Autodesk Fusion 360 part; units mm, degrees
(part 2 of 2)
sketch "Sketch1" plane through (0, 0, 0) normal (0, 0, 1) x (1, 0, 0)
  line L0 (-42.9407, 21.9767) -> (-42.9407, 26.9767)
  line L1 (-42.9407, 26.9767) -> (-52.9407, 26.9767)
  line L2 (-52.9407, 26.9767) -> (-52.9407, 31.9767)
  line L3 (-52.9407, 31.9767) -> (-47.9407, 31.9767)
  line L4 (-47.9407, 31.9767) -> (-47.9407, 41.9767)
  line L5 (-47.9407, 41.9767) -> (-52.9407, 41.9767)
  line L6 (-32.9407, 26.9767) -> (-32.9407, 21.9767)
  line L7 (-22.9407, 26.9767) -> (-32.9407, 26.9767)
  line L8 (-22.9407, 21.9767) -> (-22.9407, 26.9767)
  line L9 (-12.9407, 26.9767) -> (-12.9407, 21.9767)
  line L10 (-2.9407, 26.9767) -> (-12.9407, 26.9767)
  line L11 (-27.9407, 12.4409) -> (-27.9407, 59.643) construction
  line L12 (-59.1616, 36.9767) -> (4.5103, 36.9767) construction
  line L13 (-42.9407, 46.9767) -> (-52.9407, 46.9767)
  line L14 (-42.9407, 51.9767) -> (-42.9407, 46.9767)
  line L15 (-32.9407, 46.9767) -> (-32.9407, 51.9767)
  line L16 (-22.9407, 46.9767) -> (-32.9407, 46.9767)
  line L17 (-22.9407, 51.9767) -> (-22.9407, 46.9767)
  line L18 (-12.9407, 46.9767) -> (-12.9407, 51.9767)
  line L19 (-2.9407, 46.9767) -> (-12.9407, 46.9767)
  line L20 (-7.9407, 31.9767) -> (-7.9407, 41.9767)
  line L21 (-7.9407, 41.9767) -> (-2.9407, 41.9767)
  line L22 (-2.9407, 31.9767) -> (-7.9407, 31.9767)
  line L23 (-42.9407, 51.9767) -> (-32.9407, 51.9767)
  line L24 (-22.9407, 51.9767) -> (-12.9407, 51.9767)
  line L25 (-52.9407, 26.9767) -> (-52.9407, 31.9767)
  line L26 (-52.9407, 41.9767) -> (-52.9407, 46.9767)
  line L27 (-12.9407, 21.9767) -> (-22.9407, 21.9767)
  line L28 (-32.9407, 21.9767) -> (-42.9407, 21.9767)
  line L29 (-2.9407, 46.9767) -> (-2.9407, 41.9767)
  line L30 (-2.9407, 31.9767) -> (-2.9407, 26.9767)
  dimension "d5" = 5
  dimension "d6" = 5
  dimension "d7" = 10
  dimension "d12" = 15
  dimension "d13" = 25
  constraint horizontal L23
  constraint vertical L29
  constraint horizontal L27
  constraint vertical L25
  constraint vertical L0
  constraint horizontal L1
  constraint perpendicular L1 L2
  constraint horizontal L3
  constraint vertical L4
  constraint horizontal L5
  constraint perpendicular L11 L23
  constraint perpendicular L12 L29
  constraint symmetric L0.start L12 L14.start
  constraint symmetric L0.end L12 L13.start
  constraint symmetric L1.end L12 L13.end
  constraint symmetric L6.start L12 L15.start
  constraint symmetric L6.end L12 L15.end
  constraint symmetric L7.start L12 L16.start
  constraint symmetric L8.start L12 L17.start
  constraint symmetric L9.start L12 L18.start
  constraint symmetric L9.end L12 L18.end
  constraint symmetric L10.start L12 L19.start
  constraint symmetric L2.end L11 L22.start
  constraint symmetric L3.end L11 L20.start
  constraint symmetric L4.end L11 L20.end
  constraint symmetric L5.end L11 L21.end
  constraint collinear L23 L24
  constraint collinear L25 L26
  constraint collinear L27 L28
  constraint collinear L29 L30
  measures "d5" distance of L1.end L2.end
  measures "d6" distance of L2.end L3.end
  measures "d7" distance of L2.end L5.end
  measures "d12" distance of L12 L23
  measures "d13" distance of L11 L29
extrude "Extrude1" add sketch "Sketch1" along normal blind 5
sketch "Sketch2" plane through (0, 0, 5) normal (0, 0, 1) x (-1, 0, 0)
  line L0 (7.9407, -31.9767) -> (7.9407, -41.9767)
  line L1 (7.9407, -41.9767) -> (2.9407, -41.9767)
  line L2 (2.9407, -41.9767) -> (2.9407, -46.9767)
  line L3 (2.9407, -46.9767) -> (12.9407, -46.9767)
  line L4 (12.9407, -46.9767) -> (12.9407, -51.9767)
  line L5 (12.9407, -51.9767) -> (22.9407, -51.9767)
  line L6 (22.9407, -51.9767) -> (22.9407, -46.9767)
  line L7 (22.9407, -46.9767) -> (32.9407, -46.9767)
  line L8 (32.9407, -46.9767) -> (32.9407, -51.9767)
  line L9 (32.9407, -51.9767) -> (42.9407, -51.9767)
  line L10 (42.9407, -51.9767) -> (42.9407, -46.9767)
  line L11 (42.9407, -46.9767) -> (52.9407, -46.9767)
  line L12 (52.9407, -46.9767) -> (52.9407, -41.9767)
  line L13 (52.9407, -41.9767) -> (47.9407, -41.9767)
  line L14 (47.9407, -41.9767) -> (47.9407, -31.9767)
  line L15 (47.9407, -31.9767) -> (52.9407, -31.9767)
  line L16 (52.9407, -31.9767) -> (52.9407, -26.9767)
  line L17 (52.9407, -26.9767) -> (42.9407, -26.9767)
  line L18 (42.9407, -26.9767) -> (42.9407, -21.9767)
  line L19 (42.9407, -21.9767) -> (32.9407, -21.9767)
  line L20 (32.9407, -21.9767) -> (32.9407, -26.9767)
  line L21 (32.9407, -26.9767) -> (22.9407, -26.9767)
  line L22 (22.9407, -26.9767) -> (22.9407, -21.9767)
  line L23 (22.9407, -21.9767) -> (12.9407, -21.9767)
  line L24 (12.9407, -21.9767) -> (12.9407, -26.9767)
  line L25 (12.9407, -26.9767) -> (2.9407, -26.9767)
  line L26 (2.9407, -26.9767) -> (2.9407, -31.9767)
  line L27 (2.9407, -31.9767) -> (7.9407, -31.9767)
  line L28 (43.5617, -39.2983) -> (32.0803, -39.2983) construction
  line L29 (32.0803, -39.2983) -> (32.0803, -43.9251) construction
  line L30 (32.0803, -43.9251) -> (43.5617, -43.9251) construction
  line L31 (43.5617, -43.9251) -> (43.5617, -39.2983) construction
  dimension "d16" = 5
  text T0 "1068" font "Arial" height 5 align left top in box 11.4814 x 4.6268 at (43.5617, -39.2983) x (-1, 0) y (0, -1) spacing 1 kerned
emboss "Emboss1" depth -0.7 profiles "Sketch2" section 1 text T0 onto face at (-39.6074, 33.6433, 5)

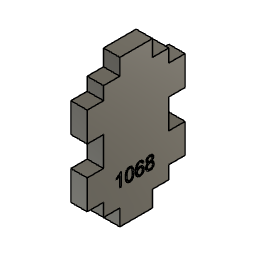
design "Housing_6"
Autodesk Fusion 360 part; units mm, degrees
sketch "Sketch1" plane through (0, 0, 0) normal (1, 0, 0) x (0, 1, 0)
  line L0 (-14.2005, 65.0328) -> (-4.2005, 65.0328)
  line L1 (-19.2005, 60.0328) -> (-19.2005, 56.0328)
  line L2 (-19.2005, 56.0328) -> (-24.2005, 56.0328)
  line L3 (-14.2005, 65.0328) -> (-14.2005, 60.0328)
  line L4 (-14.2005, 60.0328) -> (-19.2005, 60.0328)
  line L5 (-19.2005, 38.0328) -> (-24.2005, 38.0328)
  line L6 (-19.2005, 42.5328) -> (-19.2005, 38.0328)
  line L7 (-19.2005, 42.5328) -> (-19.2005, 47.0328)
  line L8 (-24.2005, 47.0328) -> (-19.2005, 47.0328)
  line L9 (-19.2005, 25.0328) -> (-19.2005, 27.5328)
  line L10 (-9.2005, 80.7683) -> (-9.2005, 14.0865) construction
  line L11 (-40.7163, 42.5328) -> (11.7648, 42.5328) construction
  line L12 (-4.2005, 60.0328) -> (0.7995, 60.0328)
  line L13 (-4.2005, 65.0328) -> (-4.2005, 60.0328)
  line L14 (0.7995, 60.0328) -> (0.7995, 56.0328)
  line L15 (0.7995, 56.0328) -> (5.7995, 56.0328)
  line L16 (5.7995, 47.0328) -> (0.7995, 47.0328)
  line L17 (0.7995, 42.5328) -> (0.7995, 47.0328)
  line L18 (0.7995, 42.5328) -> (0.7995, 38.0328)
  line L19 (0.7995, 38.0328) -> (5.7995, 38.0328)
  line L20 (-14.2005, 25.0328) -> (-19.2005, 25.0328)
  line L21 (-14.2005, 20.0328) -> (-14.2005, 25.0328)
  line L22 (-19.2005, 25.0328) -> (-19.2005, 29.0328)
  line L23 (-19.2005, 29.0328) -> (-24.2005, 29.0328)
  line L24 (-4.2005, 20.0328) -> (-4.2005, 25.0328)
  line L25 (-4.2005, 25.0328) -> (0.7995, 25.0328)
  line L26 (0.7995, 25.0328) -> (0.7995, 29.0328)
  line L27 (0.7995, 29.0328) -> (5.7995, 29.0328)
  line L28 (5.7995, 56.0328) -> (5.7995, 47.0328)
  line L29 (5.7995, 38.0328) -> (5.7995, 29.0328)
  line L30 (-4.2005, 20.0328) -> (-14.2005, 20.0328)
  line L31 (-24.2005, 29.0328) -> (-24.2005, 38.0328)
  line L32 (-24.2005, 47.0328) -> (-24.2005, 56.0328)
  line L33 (-4.2005, 65.0328) -> (-4.2005, 60.0328)
  line L34 (-4.2005, 60.0328) -> (0.7995, 60.0328)
  line L35 (0.7995, 56.0328) -> (5.7995, 56.0328)
  line L36 (0.7995, 60.0328) -> (0.7995, 56.0328)
  line L37 (5.7995, 47.0328) -> (5.7995, 56.0328)
  line L38 (5.7995, 47.0328) -> (0.7995, 47.0328)
  line L39 (0.7995, 42.5328) -> (0.7995, 47.0328)
  line L40 (-14.2005, 20.0328) -> (-14.2005, 25.0328)
  line L41 (-14.2005, 20.0328) -> (-4.2005, 20.0328)
  line L42 (-4.2005, 20.0328) -> (-4.2005, 25.0328)
  line L43 (-4.2005, 25.0328) -> (0.7995, 25.0328)
  line L44 (0.7995, 25.0328) -> (0.7995, 29.0328)
  line L45 (0.7995, 29.0328) -> (5.7995, 29.0328)
  line L46 (5.7995, 38.0328) -> (5.7995, 29.0328)
  line L47 (0.7995, 42.5328) -> (0.7995, 38.0328)
  line L48 (-19.2005, 42.5328) -> (-19.2005, 38.0328)
  line L49 (-24.2005, 38.0328) -> (-24.2005, 29.0328)
  line L50 (-19.2005, 29.0328) -> (-24.2005, 29.0328)
  line L51 (-19.2005, 25.0328) -> (-19.2005, 29.0328)
  line L52 (-14.2005, 25.0328) -> (-19.2005, 25.0328)
  dimension "d13" = 45
  dimension "d14" = 9
  dimension "d15" = 4
  dimension "d17" = 9
  dimension "d18" = 9
  constraint horizontal L0
  constraint vertical L28
  constraint horizontal L30
  constraint vertical L31
  constraint vertical L1
  constraint horizontal L2
  constraint vertical L3
  constraint horizontal L4
  constraint perpendicular L10 L30
  constraint perpendicular L11 L28
  constraint symmetric L1.end L10 L14.end
  constraint symmetric L2.end L10 L15.end
  constraint symmetric L0.start L10 L0.end
  constraint symmetric L3.end L10 L12.start
  constraint symmetric L1.start L10 L12.end
  constraint symmetric L5.start L10 L18.end
  constraint symmetric L5.end L10 L19.end
  constraint symmetric L6.start L10 L17.start
  constraint symmetric L7.end L10 L16.end
  constraint symmetric L8.start L10 L16.start
  constraint symmetric L1.end L11 L22.end
  constraint symmetric L2.end L11 L23.end
  constraint symmetric L0.start L11 L21.start
  constraint symmetric L3.end L11 L20.start
  constraint symmetric L1.start L11 L9.start
  constraint symmetric L11 L12.start L24.end
  constraint symmetric L11 L12.end L25.end
  constraint symmetric L11 L0.end L24.start
  constraint symmetric L11 L14.end L26.end
  constraint symmetric L11 L15.end L27.end
  constraint collinear L28 L29
  constraint collinear L31 L32
  constraint symmetric L6.start L11 L7.start
  constraint symmetric L7.end L11 L5.start
  constraint symmetric L11 L16.end L18.end
  constraint symmetric L11 L17.start L18.start
  measures "d13" distance of L0 L30
  measures "d14" distance of L0 L2
  measures "d15" distance of L2 L4
  measures "d17" distance of L2 L8
  measures "d18" distance of L5 L50
extrude "Extrude1" add sketch "Sketch1" along normal blind 5
sketch "Sketch2" plane through (5, 0, 0) normal (1, 0, 0) x (0, 1, 0)
  line L0 (-19.2005, 47.0328) -> (-19.2005, 38.0328)
  line L1 (-19.2005, 38.0328) -> (-24.2005, 38.0328)
  line L2 (-24.2005, 38.0328) -> (-24.2005, 29.0328)
  line L3 (-24.2005, 29.0328) -> (-19.2005, 29.0328)
  line L4 (-19.2005, 29.0328) -> (-19.2005, 25.0328)
  line L5 (-19.2005, 25.0328) -> (-14.2005, 25.0328)
  line L6 (-14.2005, 25.0328) -> (-14.2005, 20.0328)
  line L7 (-14.2005, 20.0328) -> (-4.2005, 20.0328)
  line L8 (-4.2005, 20.0328) -> (-4.2005, 25.0328)
  line L9 (-4.2005, 25.0328) -> (0.7995, 25.0328)
  line L10 (0.7995, 25.0328) -> (0.7995, 29.0328)
  line L11 (0.7995, 29.0328) -> (5.7995, 29.0328)
  line L12 (5.7995, 29.0328) -> (5.7995, 38.0328)
  line L13 (5.7995, 38.0328) -> (0.7995, 38.0328)
  line L14 (0.7995, 38.0328) -> (0.7995, 47.0328)
  line L15 (0.7995, 47.0328) -> (5.7995, 47.0328)
  line L16 (5.7995, 47.0328) -> (5.7995, 56.0328)
  line L17 (5.7995, 56.0328) -> (0.7995, 56.0328)
  line L18 (0.7995, 56.0328) -> (0.7995, 60.0328)
  line L19 (0.7995, 60.0328) -> (-4.2005, 60.0328)
  line L20 (-4.2005, 60.0328) -> (-4.2005, 65.0328)
  line L21 (-4.2005, 65.0328) -> (-14.2005, 65.0328)
  line L22 (-14.2005, 65.0328) -> (-14.2005, 60.0328)
  line L23 (-14.2005, 60.0328) -> (-19.2005, 60.0328)
  line L24 (-19.2005, 60.0328) -> (-19.2005, 56.0328)
  line L25 (-19.2005, 56.0328) -> (-24.2005, 56.0328)
  line L26 (-24.2005, 56.0328) -> (-24.2005, 47.0328)
  line L27 (-24.2005, 47.0328) -> (-19.2005, 47.0328)
  line L28 (-15.2384, 29.0856) -> (-1.443, 29.0856) construction
  line L29 (-1.443, 29.0856) -> (-1.443, 34.4691) construction
  line L30 (-1.443, 34.4691) -> (-15.2384, 34.4691) construction
  line L31 (-15.2384, 34.4691) -> (-15.2384, 29.0856) construction
  dimension "d19" = 4
  text T0 "1068" font "Arial" height 4 align left top in box 13.7954 x 5.3836 at (-15.2384, 29.0856) x (1, 0) y (0, 1) spacing 1 kerned
emboss "Emboss1" depth -0.7 profiles "Sketch2" section 1 text T0 onto face at (5, -7.5339, 51.3662)
